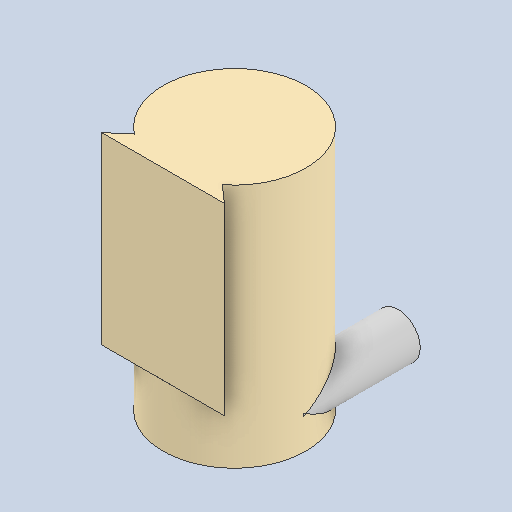
# Autodesk Inventor part: Pomp]
Saved by Autodesk Inventor 2022 (Build 260153000, 153)
## iProperties
Created: 2022-09-28
Part Number: Pomp]
Material: Ogólny
Document SubType Name: Modeling
Designer: kosak
Density: 1 g/cm^3
Appearance: Domyślna
Author: kosak
Autodesk Inventor part; units mm, degrees
ref_plane "YZ Plane" through (0, 0, 0) normal (1, 0, 0) x (0, 1, 0)
ref_plane "XZ Plane" through (0, 0, 0) normal (0, 1, 0) x (-1, 0, 0)
sketch "Szkic1" plane through (0, 0, 0) normal (0, 1, 0) x (-1, 0, 0)
  circle A0 centre (0, 0) radius 11.65
  dimension "d0" = 23.3
  constraints: 1 centre point, 1 coincident
  measures "d0" diameter of A0
extrude "Wyciągnięcie proste1" add sketch "Szkic1" along normal blind 40
sketch "Szkic2" plane through (0, 40, 0) normal (0, 1, 0) x (1, 0, 0)
  circle A0 centre (0, 0) radius 11.65 projected
  line L0 (0, -11.65) -> (-10, -11.65)
  arc A1 (-7.185, -9.1705) -> (0, -11.65) centre (0, 0) ccw
  line L1 (0, -11.65) -> (-7.185, -11.65)
  line L2 (0, -9.1705) -> (-7.185, -9.1705)
  line L3 (0, -11.65) -> (0, -5.8216)
  line L4 (-10, -11.65) -> (-7.185, -9.1705)
  line L5 (0, -11.65) -> (10, -11.65)
  line L6 (0, -9.1705) -> (7.185, -9.1705)
  line L7 (10, -11.65) -> (7.185, -9.1705)
  dimension "d3" = 10
  dimension "d6" = 7.185
  constraints: 16 end point, 4 point on circle, 2 horizontal, 2 point on line, 2 symmetric about line, 2 tangent, 1 centre point, 1 concentric, 1 vertical
  measures "d3" distance of L0.start L0.end
  measures "d6" distance of L2.end L2.start
extrude "Wyciągnięcie proste2" add sketch "Szkic2" against normal blind 30 contours A0 L0 L4 | L7 L5 A0
ref_plane "Płaszczyzna konstrukcyjna1" through (0, 0, -11.65) normal (0, 0, 1) x (1, 0, 0)
sketch "Szkic3" plane through (0, 0, -11.65) normal (0, 0, 1) x (1, 0, 0)
  circle A0 centre (8.025, 5.275) radius 3.625
  line L0 (11.65, 0) -> (-11.65, 0) projected
  line L1 (11.65, 8.9) -> (-11.65, 8.9)
  circle A1 centre (8.025, 5.275) radius 2
  point P0 (0, 0)
  dimension "d10" = 8.9
  dimension "d11" = 4
  constraints: 2 centre point, 2 end point, 1 coincident, 1 parallel, 1 tangent
  measures "d10" distance between parallel lines of L0 L1
  measures "d11" diameter of A1
extrude "Wyciągnięcie proste3" add sketch "Szkic3" along normal blind 12 and the other way blind 7 contours A0 | A1
